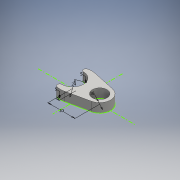
# Autodesk Inventor part: 240412_sketch4
Saved by Autodesk Inventor 2016 (Build 200138000, 138)
## iProperties
Created: 2024-04-12
Part Number: 240412_sketch4
Material: 일반
Document SubType Name: Modeling
Designer: pc
Density: 1 g/cm^3
Appearance: 기본값
Author: pc
Autodesk Inventor part; units mm, degrees
ref_plane "YZ Plane" through (0, 0, 0) normal (1, 0, 0) x (0, 1, 0)
ref_plane "XZ Plane" through (0, 0, 0) normal (0, 1, 0) x (-1, 0, 0)
ref_plane "XY Plane" through (0, 0, 0) normal (0, 0, 1) x (1, 0, 0)
sketch "스케치1" plane through (0, 0, 0) normal (0, 0, 1) x (1, 0, 0)
  line L0 (0, 41.7955) -> (0, -35.3319)
  line L1 (-51.4236, 0) -> (57.1089, 0)
  arc A0 (-13.077, -11.9993) -> (-13.077, 11.9993) centre (-13.2063, 0) ccw
  circle A1 centre (16.7937, 0) radius 8
  line L2 (19.3321, 11.7284) -> (-5.5044, 17.104)
  line L3 (19.3321, -11.7284) -> (-5.5044, -17.104)
  arc A2 (-13.6907, 16.9157) -> (-13.077, 11.9993) centre (-13.0501, 14.4992) ccw
  arc A3 (-13.077, -11.9993) -> (-13.6907, -16.9157) centre (-13.0501, -14.4992) ccw
  arc A4 (19.3321, -11.7284) -> (19.3321, 11.7284) centre (16.7937, 0) ccw
  arc A5 (-5.5044, 17.104) -> (-13.6907, 16.9157) centre (-9.2063, 0) ccw
  arc A6 (-13.6907, -16.9157) -> (-5.5044, -17.104) centre (-9.2063, 0) ccw
  point P0 (0, 0)
  dimension "d1" = 24
  dimension "d4" = 30
  dimension "d8" = 16
  dimension "d9" = 4
  dimension "d10" = 5
  dimension "d11" = 5
  constraints: 12 point on circle, 8 end point, 7 centre point, 6 tangent, 3 point on line, 1 coincident, 1 horizontal, 1 vertical
  measures "d1" diameter of A0
  measures "d4" distance of A0.centre A4.centre
  measures "d8" diameter of A1
  measures "d9" distance of A5.centre A0.centre
  measures "d10" diameter of A2
  measures "d11" diameter of A3
extrude "돌출1" add sketch "스케치1" along normal blind 10 contours L2 A4 L1 A1 L0 | L0 L1 A0 A2 A5 L2 | L1 A1 A4 L3 L0 | L0 L3 A6 A3 A0 L1
